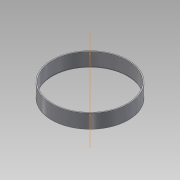
# Autodesk Inventor part: bucket
Saved by Autodesk Inventor 2019.3 (Build 233278000, 278)
## iProperties
Created: 2019-03-03
Part Number: bucket
Material: ABS Plastic
Document SubType Name: Modeling
Designer: WW
Density: 1.06 g/cm^3
Appearance: Smooth - White
Author: WW
Autodesk Inventor part; units mm, degrees
ref_plane "XZ Plane" through (0, 0, 0) normal (0, 1, 0) x (-1, 0, 0)
ref_plane "XY Plane" through (0, 0, 0) normal (0, 0, 1) x (1, 0, 0)
sketch "Sketch1" plane through (0, 0, 0) normal (0, 0, 1) x (1, 0, 0)
  line L0 (0, 0) -> (0, -20.7931)
  line L1 (117, 0) -> (117, 43)
  line L2 (117, 43) -> (114.25, 43)
  line L3 (114.25, 43) -> (114.25, 3)
  line L4 (114.25, 3) -> (116, 3)
  line L5 (116, 3) -> (116, 0)
  line L6 (116, 0) -> (117, 0)
  dimension "d1" = 234
  dimension "d2" = 228.5
  dimension "d6" = 1
  dimension "d7" = 3
  constraints: 14 end point, 4 perpendicular, 1 horizontal, 1 horizontal alignment, 1 vertical
  measures "d1" diameter of L1 L0
  measures "d2" diameter of L3 L0
  measures "d6" distance between parallel lines of L1 L5
  measures "d7" distance between parallel lines of L6 L4
revolve "Revolution1" add sketch "Sketch1" angle 360 about axis through (0, 0, 0) along (0, -1, 0)
ref_plane "Work Plane1" through (0, 0, 0) normal (0.7071, 0, -0.7071) x (0, 1, 0)
sketch "Sketch2" plane through (0, 0, 0) normal (0.7071, 0, -0.7071) x (0, 1, 0)
  circle A0 centre (36.5, 0) radius 2.5
  line L0 (43, 117) -> (43, -117) construction
  point P0 (0, 0)
  point P1 (43, 0)
  dimension "d9" = 5
  dimension "d10" = 6.5
  constraints: 1 centre point, 1 horizontal alignment, 1 midpoint
  measures "d9" diameter of A0
  measures "d10" distance from line of L0 A0.centre
extrude "Extrusion1" cut sketch "Sketch2" along normal through all both and the other way through all
pattern_circular "Circular Pattern1" count 4 over 360 about axis through (0, 21.5, 0) along (0, -1, 0) of "Extrusion1"
body "Solid1"
